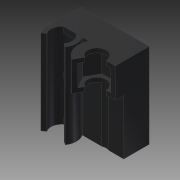
# Autodesk Inventor part: X_left
Saved by Autodesk Inventor 2013 (Build 170138000, 138)
## iProperties
Created: 2014-01-22
Part Number: X_left
Material: Generic
Document SubType Name: Modeling
Designer: Masta
Density: 1 g/cm^3
Author: Masta
Autodesk Inventor part; units mm, degrees
ref_plane "YZ Plane" through (0, 0, 0) normal (1, 0, 0) x (0, 1, 0)
ref_plane "XZ Plane" through (0, 0, 0) normal (0, 1, 0) x (-1, 0, 0)
ref_plane "XY Plane" through (0, 0, 0) normal (0, 0, 1) x (1, 0, 0)
sketch "Sketch1" plane through (0, 0, 0) normal (0, 0, 1) x (1, 0, 0)
  arc A0 (6.1436, -4.3018) -> (4.5, 6) centre (0, 0) ccw
  line L0 (0, 0) -> (25, 0) construction
  line L1 (15.1273, 0) -> (18.5914, 6)
  line L2 (20.0637, 8.55) -> (29.9363, 8.55)
  line L3 (29.9363, 8.55) -> (31.4086, 6)
  line L4 (29.9363, -8.55) -> (20.0637, -8.55) construction
  line L5 (20.0637, -8.55) -> (15.1273, 0)
  line L6 (-22.0744, 26) -> (39.9256, 26) construction
  line L7 (-10.5, 24) -> (38, 24)
  line L8 (38, 24) -> (38, 6)
  circle A1 centre (25, 0) radius 5 construction
  line L9 (38, 6) -> (31.4086, 6)
  line L10 (-10.5, 6) -> (-10.5, 24)
  line L11 (38, 6) -> (38, 0)
  line L12 (38, 0) -> (25, 0) construction
  arc A2 (13.4674, 6) -> (18.5, -11.2583) centre (25, 0) ccw
  line L13 (-10.5, 6) -> (-10.5, 0)
  arc A3 (-10.5, 0) -> (-8.6011, -6.0226) centre (0, 0) ccw
  line L14 (38, 15) -> (-10.5, 15) construction
  line L15 (-10.5, 19) -> (38, 19) construction
  line L16 (38, 11) -> (-10.5, 11) construction
  line L17 (6.1436, -4.3018) -> (8.6011, -6.0226)
  line L18 (0, 0) -> (0, -10.5) construction
  line L19 (-6.1436, -4.3018) -> (-8.6011, -6.0226)
  arc A4 (-8.6011, -6.0226) -> (8.6011, -6.0226) centre (0, 0) ccw construction
  arc A5 (8.6011, -6.0226) -> (8.6168, 6) centre (0, 0) ccw
  arc A6 (-6.1436, -4.3018) -> (6.1436, -4.3018) centre (0, 0) ccw construction
  line L20 (-4.5, 6) -> (-10.5, 6)
  line L21 (4.5, 6) -> (-4.5, 6)
  line L22 (-4.5, 6) -> (4.5, 6) construction
  line L23 (34.8727, 0) -> (29.9363, -8.55) construction
  arc A7 (18.5, -11.2583) -> (38, 0) centre (25, 0) ccw construction
  arc A8 (21.75, -5.6292) -> (31.5, 0) centre (25, 0) ccw
  line L24 (18.5914, 6) -> (20.0637, 8.55)
  line L25 (31.4086, 6) -> (34.8727, 0)
  line L26 (15.1273, 0) -> (18.5, 0) construction
  line L27 (22.5, 6) -> (22.5, 6) construction
  line L28 (22.5, 6) -> (8.6168, 6)
  line L29 (31.4086, 6) -> (22.5, 6)
  line L30 (6.1436, -4.3018) -> (0, 0) construction
  line L31 (8.6168, 6) -> (4.5, 6)
  arc A9 (4.5, 6) -> (-6.1436, -4.3018) centre (0, 0) ccw
  circle A10 centre (0, 0) radius 4 construction
  line L32 (34.8727, 0) -> (38, 0)
  line L33 (20.0637, -8.55) -> (18.5, -11.2583)
  line L34 (25, 0) -> (20.0637, -8.55) construction
  line L35 (31.5, 0) -> (34.8727, 0)
  line L36 (20.0637, -8.55) -> (21.75, -5.6292)
  arc A11 (18.5, 0) -> (21.75, -5.6292) centre (25, 0) ccw
  arc A12 (31.5, 0) -> (27.5, 6) centre (25, 0) ccw
  arc A13 (27.5, 6) -> (22.5, 6) centre (25, 0) ccw
  arc A14 (22.5, 6) -> (18.5, 0) centre (25, 0) ccw
  dimension "d0" = 15
  dimension "d1" = 25
  dimension "d2" = 17.1
  dimension "d3" = 26
  dimension "d4" = 2
  dimension "d5" = 18
  dimension "d6" = 10
  dimension "d7" = 13
  dimension "d8" = 3
  dimension "d9" = 8
  dimension "d10" = 110
  dimension "d11" = 6
  dimension "d14" = 13
  dimension "d26" = 8
  constraints: 74 end point, 40 point on circle, 18 perpendicular, 15 centre point, 13 point on line, 9 coincident, 7 collinear, 5 parallel, 3 midpoint, 3 tangent, 2 symmetric about line, 1 concentric, 1 horizontal, 13 other
  measures "d0" diameter of A0
  measures "d1" distance of L0.start L0.end
  measures "d2" distance between parallel lines of L2 L4
  measures "d3" distance between parallel lines of L6 L0
  measures "d4" distance between parallel lines of L6 L7
  measures "d5" distance of L7.end L8.end
  measures "d6" diameter of A1
  measures "d7" radius of A2
  measures "d8" radial gap between concentric circles of A0 A3
  measures "d9" distance between parallel lines of L15 L16
  measures "d10" angle of L17 L19
  measures "d11" distance between parallel lines of L22 L0
  measures "d14" diameter of A8
  measures "d26" diameter of A10
extrude "Extrusion1" add sketch "Sketch1" against normal blind 60 contours A0 L31 A5 L17 | A9 L20 L10 L7 L8 L9 L3 L2 L24 L28 L31 | A9 L19 A3 L13 L20 | L24 L2 L3 L29 A13 L28
extrude "Extrusion2" add sketch "Sketch1" against normal blind 21 contours L28 L1 L5 L33 A2 | L11 L32 L25 L9
extrude "Extrusion3" add sketch "Sketch1" against normal blind 3 contours A9 L20 L10 L7 L8 L9 L3 L2 L24 L28 L31 | L28 L1 L5 L33 A2 | L28 A14 A11 L36 L5 L1 | L29 L25 L35 A12
pattern_linear "Rectangular Pattern1" count 2 spacing 18 along (0, 0, -1) of "Extrusion3"
extrude "Extrusion4" cut sketch "Sketch1" against normal up to surface (15 mm away) from surface at -3 contours L24 L2 L3 L29 A13 L28
extrude "Extrusion5" add sketch "Sketch1" against normal blind 4 contours L21 A9
pattern_linear "Rectangular Pattern2" count 3 spacing 28 along (0, 0, -1) of "Extrusion5"
body "Solid1"
